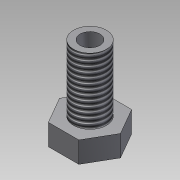
# Autodesk Inventor part: Pusher.Bolt
Saved by Autodesk Inventor 2011 (Build 150239000, 239)
## iProperties
Created: 2011-04-01
Part Number: Pusher.Bolt
Document SubType Name: Modeling
Designer: Rob
Density: 1 g/cm^3
Author: Rob
Autodesk Inventor part; units mm, degrees
ref_plane "YZ Plane" through (0, 0, 0) normal (1, 0, 0) x (0, 1, 0)
ref_plane "XZ Plane" through (0, 0, 0) normal (0, 1, 0) x (-1, 0, 0)
ref_plane "XY Plane" through (0, 0, 0) normal (0, 0, 1) x (1, 0, 0)
sketch "Sketch1" plane through (0, 0, 0) normal (0, 0, 1) x (1, 0, 0)
  circle A0 centre (0, 0) radius 8
  line L0 (-8, -8) -> (8, -8)
  line L1 (2.9282, -10.9282) -> (10.9282, 2.9282)
  line L2 (10.9282, -2.9282) -> (2.9282, 10.9282)
  line L3 (8, 8) -> (-8, 8)
  line L4 (-2.9282, 10.9282) -> (-10.9282, -2.9282)
  line L5 (-10.9282, 2.9282) -> (-2.9282, -10.9282)
  line L6 (-4.6188, -8) -> (4.6188, -8)
  line L7 (9.2376, 0) -> (4.6188, -8)
  line L8 (4.6188, 8) -> (9.2376, 0)
  line L9 (4.6188, 8) -> (-4.6188, 8)
  line L10 (-4.6188, 8) -> (-9.2376, 0)
  line L11 (-9.2376, 0) -> (-4.6188, -8)
  dimension "d0" = 16
  dimension "d3" = 360
  constraints: 24 end point, 11 point on line, 3 collinear, 1 centre point, 1 coincident, 1 horizontal, 19 other
  measures "d0" diameter of A0
extrude "Extrusion1" add sketch "Sketch1" along normal blind 6.4
sketch "Sketch2" plane through (0, 0, 6.4) normal (0, 0, 1) x (1, 0, 0)
  circle A0 centre (0, 0) radius 5
  dimension "d7" = 10
  constraints: 1 centre point, 1 coincident
  measures "d7" diameter of A0
extrude "Extrusion2" add sketch "Sketch2" along normal blind 20
thread "Thread1" size "M10x1.5" class "6g" standard "ANSI Metric M Profile" full length
sketch "Sketch3" plane through (0, 0, 0) normal (0, 0, -1) x (-1, 0, 0)
  circle A0 centre (0, 0) radius 3
  dimension "d12" = 6
  constraints: 1 centre point, 1 coincident
  measures "d12" diameter of A0
extrude "Extrusion3" cut sketch "Sketch3" against normal through all
body "Solid1"
